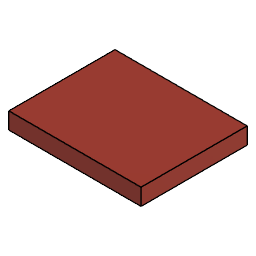
przetwornica (Autodesk Fusion 360 design; units mm, degrees)
part number: 2025-11-21-11-59-02-291
part number: 2025-11-29-20-27-12-206
Autodesk Fusion 360 part; units mm, degrees
sketch "Szkic1" plane through (0, 0, 0) normal (0, 0, 1) x (1, 0, 0)
  line L0 (0, 0) -> (12.7, 0)
  line L1 (12.7, 0) -> (12.7, 10.2)
  line L2 (12.7, 10.2) -> (0, 10.2)
  line L3 (0, 10.2) -> (0, 0)
  dimension "d1" = 12.7
  dimension "d2" = 10.2
  constraint horizontal L0
  constraint vertical L1
  constraint horizontal L2
  constraint vertical L3
  constraint coincident L0.start L3.end
  measures "d1" distance of L0.start L0.end
  measures "d2" distance of L0.start L2.end
extrude "Wyciągnięcie proste1" add sketch "Szkic1" along normal blind 1.6 makes body 1
copy_body "Bryła->Komponent1" bodies 1 removing the originals makes body 2 in component "Component"
component "Component" placed x (1, 0, 0) y (0, 1, 0) z (0, 0, 1) at (0, 0, 0)
